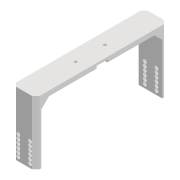
# Autodesk Inventor part: Led_frame_2
Saved by Autodesk Inventor 2020 (Build 240168000, 168)
## iProperties
Created: 2021-06-21
Part Number: Led_frame_2
Material: Generic
Document SubType Name: Modeling
Designer: CDT
Density: 1 g/cm^3
Appearance: Default
Author: CDT
Autodesk Inventor part; units mm, degrees
ref_plane "YZ Plane" through (0, 0, 0) normal (1, 0, 0) x (0, 1, 0)
ref_plane "XZ Plane" through (0, 0, 0) normal (0, 1, 0) x (-1, 0, 0)
ref_plane "XY Plane" through (0, 0, 0) normal (0, 0, 1) x (1, 0, 0)
sketch "Sketch1" plane through (0, 0, 0) normal (0, 0, 1) x (1, 0, 0)
  line L0 (6.9517, -19.3843) -> (18.9517, -19.3843)
  line L1 (18.9517, -19.3843) -> (18.9517, 40.6157)
  line L2 (18.9517, 40.6157) -> (6.9517, 40.6157)
  line L3 (6.9517, 40.6157) -> (6.9517, -19.3843)
  line L4 (18.9517, -19.3843) -> (30.9517, -19.3843)
  line L5 (30.9517, -19.3843) -> (30.9517, 40.6157)
  line L6 (30.9517, 40.6157) -> (18.9517, 40.6157)
  line L7 (18.9517, 40.6157) -> (18.9517, -19.3843)
  point P0 (0, 0)
  dimension "d0" = 12
  dimension "d1" = 60
  dimension "d2" = 12
  dimension "d3" = 60
  dimension "d7" = 24
  constraints: 16 end point, 4 parallel, 2 horizontal, 2 perpendicular, 1 collinear
  measures "d0" distance of L2.end L1.end
  measures "d1" distance of L1.end L0.end
  measures "d2" distance of L6.end L5.end
  measures "d3" distance of L5.end L4.end
  measures "d7" distance between parallel lines of L5 L3
extrude "Extrusion1" add sketch "Sketch1" along normal blind 5.5
sketch "Sketch3" plane through (6.9517, 40.6157, 0) normal (0, 1, 0) x (1, 0, 0)
  line L0 (0, 0) -> (0, -5.5) projected
  line L1 (0, -5.5) -> (24, -5.5)
  line L2 (24, -5.5) -> (24, 129.5)
  line L3 (24, 129.5) -> (0, 129.5)
  line L4 (0, 129.5) -> (0, -5.5)
  point P0 (-6.9517, 0)
  point P1 (0, 0)
  point P2 (24, -5.5)
  dimension "d16" = 24
  dimension "d17" = 135
  dimension "d139" = 24
  constraints: 8 end point, 2 parallel, 1 horizontal, 1 perpendicular
  measures "d16" distance of L3.end L2.end
  measures "d17" distance of L2.end L1.end
  measures "d139" distance of L0.end point (24, -5.5)
extrude "Extrusion3" add sketch "Sketch3" along normal blind 5
sketch "Sketch4" plane through (6.9517, 40.6157, 0) normal (0, -1, 0) x (1, 0, 0)
  line L0 (24, -129.5) -> (12, -129.5)
  line L1 (12, -129.5) -> (12, -124)
  line L2 (12, -124) -> (24, -124)
  line L3 (24, -124) -> (24, -129.5)
  line L4 (0, -129.5) -> (0, 0) projected
  line L5 (0, -129.5) -> (12, -129.5)
  line L6 (12, -129.5) -> (12, -124)
  line L7 (12, -124) -> (0, -124)
  line L8 (0, -124) -> (0, -129.5)
  point P0 (-6.9517, 0)
  point P1 (0, -124)
  dimension "d20" = 12
  dimension "d21" = 5.5
  dimension "d22" = 12
  dimension "d23" = 5.5
  constraints: 16 end point, 4 parallel, 2 horizontal, 2 perpendicular
  measures "d20" distance of L1.end L2.end
  measures "d21" distance of L0.end L1.end
  measures "d22" distance of L7.end L6.end
  measures "d23" distance of L6.end L5.end
extrude "Extrusion4" add sketch "Sketch4" along normal up to surface (60 mm away)
ref_plane "Work Plane1" through (-20.0483, 0.6157, -135) normal (0, 0, -1) x (0, 1, 0)
chamfer "Chamfer6" distance 8 angle 45 2 edges at (18.9517, 40.6157, 0) (18.9517, 40.6157, -124)
sketch "Sketch8" plane through (6.9517, 40.6157, 0) normal (0, -1, 0) x (1, 0, 0)
  circle A0 centre (12, -62) radius 10.5
  line L0 (24, -57) -> (0, -57)
  line L1 (0, -57) -> (0, -68)
  line L2 (0, -68) -> (24, -68)
  line L3 (24, -68) -> (24, -57)
  line L4 (24, -129.5) -> (0, -129.5) projected
  line L5 (0, 5.5) -> (24, 5.5) projected
  line L6 (0, -116) -> (0, -8) projected
  line L7 (24, -8) -> (24, -116) projected
  point P0 (-6.9517, 0)
  point P1 (47, -8)
  point P2 (3.3832, -68)
  point P3 (2.7669, -57)
  point P4 (20.6168, -68)
  point P5 (21.2331, -57)
  dimension "d84" = 21
  dimension "d141" = 6
  dimension "d142" = 5
  dimension "d162" = 135
  dimension "d163" = 67.5
  dimension "d164" = 24
  dimension "d165" = 12
  dimension "d166" = 0
  dimension "d167" = 0
  constraints: 8 end point, 2 parallel, 1 centre point, 1 horizontal, 1 perpendicular
  measures "d84" diameter of A0
  measures "d141" distance from line of A0.centre L2
  measures "d142" distance from line of L0 A0.centre
  measures "d162" distance between parallel lines of L4 L5
  measures "d163" distance from line of L4 A0.centre
  measures "d164" distance between parallel lines of L6 L7
  measures "d165" distance from line of L6 A0.centre
  measures "d166" distance between parallel lines of L6 L1
  measures "d167" distance between parallel lines of L7 L3
extrude "Extrusion8" cut sketch "Sketch8" against normal blind 2.5
sketch "Sketch9" plane through (0, 0, 5.5) normal (0, 0, 1) x (1, 0, 0)
  circle A0 centre (12.9517, -15.3843) radius 2
  circle A1 centre (12.9517, -11.3843) radius 2
  circle A2 centre (12.9517, -7.3843) radius 2
  circle A3 centre (12.9517, -3.3843) radius 2
  circle A4 centre (12.9517, 0.6157) radius 2
  line L0 (6.9517, -19.3843) -> (30.9517, -19.3843) projected
  line L1 (6.9517, -19.3843) -> (6.9517, 45.6157) projected
  circle A5 centre (12.9517, 4.6157) radius 2
  line L2 (30.9517, -19.3843) -> (30.9517, 45.6157) projected
  circle A6 centre (24.9517, -15.3843) radius 2
  circle A7 centre (24.9517, -11.3843) radius 2
  circle A8 centre (24.9517, -3.3843) radius 2
  circle A9 centre (24.9517, 4.6157) radius 2
  circle A10 centre (24.9517, 0.6157) radius 2
  circle A11 centre (24.9517, -7.3843) radius 2
  point P0 (0, 0)
  point P1 (10.9517, 19.6157)
  point P2 (18.9517, 40.6157)
  dimension "d96" = 4
  dimension "d97" = 4
  dimension "d98" = 4
  dimension "d99" = 4
  dimension "d101" = 4
  dimension "d104" = 4
  dimension "d105" = 6
  dimension "d106" = 6
  dimension "d107" = 4
  dimension "d108" = 6
  dimension "d109" = 4
  dimension "d110" = 6
  dimension "d111" = 4
  dimension "d112" = 4
  dimension "d113" = 6
  dimension "d116" = 4
  dimension "d117" = 6
  dimension "d118" = 4
  dimension "d121" = 4
  dimension "d122" = 4
  dimension "d123" = 4
  dimension "d124" = 4
  dimension "d125" = 4
  dimension "d126" = 4
  dimension "d127" = 6
  dimension "d128" = 6
  dimension "d129" = 6
  dimension "d130" = 6
  dimension "d131" = 6
  dimension "d132" = 6
  dimension "d134" = 4
  dimension "d135" = 4
  dimension "d136" = 4
  dimension "d137" = 4
  dimension "d138" = 4
  dimension "d168" = 4
  dimension "d169" = 12
  constraints: 12 centre point, 1 other
  measures "d96" diameter of A0
  measures "d97" diameter of A1
  measures "d98" diameter of A2
  measures "d99" diameter of A3
  measures "d101" diameter of A4
  measures "d104" distance from line of L0 A0.centre
  measures "d107" distance of A0.centre A1.centre
  measures "d109" distance of A1.centre A2.centre
  measures "d111" distance of A2.centre A3.centre
  measures "d112" distance of A3.centre A4.centre
  measures "d116" diameter of A5
  measures "d118" distance of A4.centre A5.centre
  measures "d121" diameter of A6
  measures "d122" diameter of A7
  measures "d123" diameter of A8
  measures "d124" diameter of A9
  measures "d125" diameter of A10
  measures "d126" diameter of A11
  measures "d127" distance from line of L2 A6.centre
  measures "d128" distance from line of L2 A7.centre
  measures "d129" distance from line of L2 A11.centre
  measures "d130" distance from line of L2 A8.centre
  measures "d131" distance from line of L2 A10.centre
  measures "d132" distance from line of L2 A9.centre
  measures "d134" distance of A6.centre A7.centre
  measures "d135" distance of A7.centre A11.centre
  measures "d136" distance of A11.centre A8.centre
  measures "d137" distance of A8.centre A10.centre
  measures "d138" distance of A10.centre A9.centre
  measures "d168" distance from line of L0 A6.centre
  measures "d169" distance of A9.centre A5.centre
extrude "Extrusion9" cut sketch "Sketch9" against normal up to surface (135 mm away)
sketch "Sketch10" plane through (6.9517, 40.6157, 0) normal (0, -1, 0) x (1, 0, 0)
  circle A0 centre (12, -47) radius 1.5
  circle A1 centre (12, -77) radius 1.5
  line L0 (21.2331, -57) -> (24, -57) projected
  line L1 (24, -68) -> (20.6168, -68) projected
  line L2 (0, -57) -> (0, -8) projected
  line L3 (24, -8) -> (24, -57) projected
  line L4 (24, -68) -> (24, -116) projected
  point P0 (-6.9517, 0)
  dimension "d143" = 3
  dimension "d144" = 3
  dimension "d145" = 30
  dimension "d146" = 10
  dimension "d147" = 9
  dimension "d170" = 24
  dimension "d171" = 12
  dimension "d172" = 12
  constraints: 2 centre point
  measures "d143" diameter of A0
  measures "d144" diameter of A1
  measures "d145" distance of A1.centre A0.centre
  measures "d146" distance from line of L0 A0.centre
  measures "d147" distance from line of A1.centre L1
  measures "d170" distance between parallel lines of L2 L3
  measures "d171" distance from line of L3 A0.centre
  measures "d172" distance from line of L4 A1.centre
extrude "Extrusion10" cut sketch "Sketch10" against normal blind 10
sketch "Sketch11" plane through (6.9517, 40.6157, 0) normal (0, -1, 0) x (1, 0, 0)
  circle A0 centre (12, -47) radius 1.5 projected
  circle A1 centre (12, -47) radius 1.5
  circle A2 centre (12, -47) radius 4.5
  circle A3 centre (12, -77) radius 1.5 projected
  circle A4 centre (12, -77) radius 1.5
  circle A5 centre (12, -77) radius 4.5
  point P0 (-6.9517, 0)
  dimension "d154" = 3
  dimension "d155" = 9
  dimension "d156" = 9
  constraints: 4 centre point, 4 coincident
  measures "d154" diameter of A1
  measures "d155" diameter of A2
  measures "d156" diameter of A5
extrude "Extrusion11" [suppressed]
chamfer "Chamfer7" [suppressed]
chamfer "Chamfer8" distance 3.8 angle 45 4 edges at (30.9517, 13.1157, -129.5) (6.9517, 13.1157, -129.5) (30.9517, 13.1157, 5.5) (6.9517, 13.1157, 5.5)
equation "\"d1\" = d3"
equation "\"d23\" = d21"
body "Solid1"
